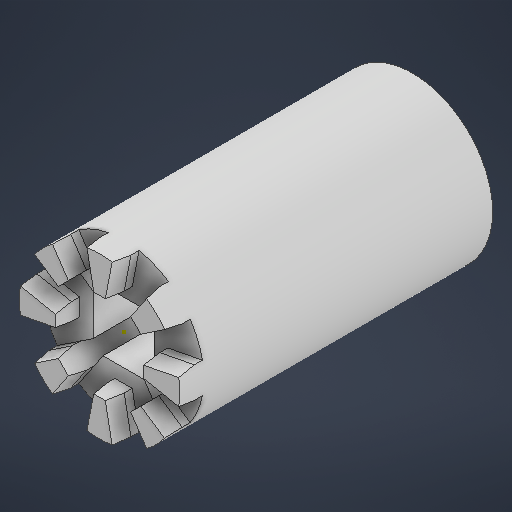
# Autodesk Inventor part: деталь вв
Saved by Autodesk Inventor 2025 (Build 290162000, 162)
## iProperties
Created: 2024-11-26
Part Number: деталь вв
Material: Типовые
Document SubType Name: Modeling
Designer: Phantom
Density: 1 g/cm^3
Appearance: По умолчанию
Author: Phantom
Autodesk Inventor part; units mm, degrees
ref_plane "YZ Plane" through (0, 0, 0) normal (1, 0, 0) x (0, 1, 0)
ref_plane "XZ Plane" through (0, 0, 0) normal (0, 1, 0) x (-1, 0, 0)
ref_plane "XY Plane" through (0, 0, 0) normal (0, 0, 1) x (1, 0, 0)
sketch "Эскиз1" plane through (0, 0, 0) normal (0, 0, 1) x (1, 0, 0)
  circle A0 centre (0, 0) radius 10
  line L0 (-3.8095, 3.8095) -> (3.8095, 3.8095)
  line L1 (3.8095, 3.8095) -> (3.8095, -3.8095)
  line L2 (3.8095, -3.8095) -> (-3.8095, -3.8095)
  line L3 (-3.8095, -3.8095) -> (-3.8095, 3.8095)
  line L4 (-3.8095, 3.8095) -> (3.8095, -3.8095) construction
  line L5 (3.8095, 3.8095) -> (-3.8095, -3.8095) construction
  dimension "d0" = 20
  constraints: 12 end point, 2 midpoint, 2 parallel, 1 centre point, 1 coincident, 1 horizontal, 1 perpendicular
  measures "d0" diameter of A0
extrude "Выдавливание1" add sketch "Эскиз1" along normal blind 36
sketch "Эскиз2" plane through (0, 0, 36) normal (0, 0, 1) x (1, 0, 0)
  line L0 (-3.8095, 3.8095) -> (3.8095, 3.8095) projected
  circle A0 centre (0, 0) radius 10 projected
  line L1 (9.8151, 1.914) -> (5.5, 1.0725)
  line L2 (5.5, -1.0775) -> (9.8135, -1.9225)
  line L3 (5.5, 0) -> (5.5, 1.0725)
  line L4 (5.5, 1.0725) -> (5.5, -1.0775)
  line L5 (5.587, 8.2937) -> (3.1307, 4.6475)
  line L6 (4.651, 3.1272) -> (8.2986, 5.5797)
  line L7 (3.8891, 3.8891) -> (3.1307, 4.6475)
  line L8 (3.1307, 4.6475) -> (4.651, 3.1272)
  line L9 (-1.914, 9.8151) -> (-1.0725, 5.5)
  line L10 (1.0775, 5.5) -> (1.9225, 9.8135)
  line L11 (0, 5.5) -> (-1.0725, 5.5)
  line L12 (-1.0725, 5.5) -> (1.0775, 5.5)
  line L13 (-8.2937, 5.587) -> (-4.6475, 3.1307)
  line L14 (-3.1272, 4.651) -> (-5.5797, 8.2986)
  line L15 (-3.8891, 3.8891) -> (-4.6475, 3.1307)
  line L16 (-4.6475, 3.1307) -> (-3.1272, 4.651)
  line L17 (-9.8151, -1.914) -> (-5.5, -1.0725)
  line L18 (-5.5, 1.0775) -> (-9.8135, 1.9225)
  line L19 (-5.5, 0) -> (-5.5, -1.0725)
  line L20 (-5.5, -1.0725) -> (-5.5, 1.0775)
  line L21 (-5.587, -8.2937) -> (-3.1307, -4.6475)
  line L22 (-4.651, -3.1272) -> (-8.2986, -5.5797)
  line L23 (-3.8891, -3.8891) -> (-3.1307, -4.6475)
  line L24 (-3.1307, -4.6475) -> (-4.651, -3.1272)
  line L25 (1.914, -9.8151) -> (1.0725, -5.5)
  line L26 (-1.0775, -5.5) -> (-1.9225, -9.8135)
  line L27 (0, -5.5) -> (1.0725, -5.5)
  line L28 (1.0725, -5.5) -> (-1.0775, -5.5)
  line L29 (8.2937, -5.587) -> (4.6475, -3.1307)
  line L30 (3.1272, -4.651) -> (5.5797, -8.2986)
  line L31 (3.8891, -3.8891) -> (4.6475, -3.1307)
  line L32 (4.6475, -3.1307) -> (3.1272, -4.651)
  dimension "d36" = 360
  constraints: 64 end point, 2 point on circle, 73 other
extrude "Выдавливание2" add sketch "Эскиз2" along normal blind 3 contours A0 L2 L4 L3 L1 | L6 L8 L7 L5 A0 | A0 L30 L32 L31 L29 | L10 L12 L11 L9 A0 | A0 L26 L28 L27 L25 | L14 L16 L15 L13 A0 | A0 L22 L24 L23 L21 | L18 L20 L19 L17 A0
chamfer "Фаска1" distance 2 angle 10 1 edges at (4.3588, 6.4706, 39) measured on face at (4.3588, 6.4706, 38.5)
chamfer "Фаска2" distance 2 angle 10 1 edges at (6.4748, 4.3535, 39) measured on face at (6.4748, 4.3535, 38.5)
chamfer "Фаска3" distance 2 angle 10 1 edges at (7.6576, 1.4932, 39) measured on face at (7.6576, 1.4932, 38.5)
chamfer "Фаска4" distance 2 angle 10 1 edges at (7.6567, -1.5, 39) measured on face at (7.6567, -1.5, 38.5)
chamfer "Фаска5" distance 2 angle 10 1 edges at (6.4706, -4.3588, 39) measured on face at (6.4706, -4.3588, 38.5)
chamfer "Фаска6" distance 2 angle 10 1 edges at (4.3535, -6.4748, 39) measured on face at (4.3535, -6.4748, 38.5)
chamfer "Фаска7" distance 2 angle 10 1 edges at (-1.5, -7.6567, 39) measured on face at (-1.5, -7.6567, 38.5)
chamfer "Фаска8" distance 2 angle 10 1 edges at (1.4932, -7.6576, 39) measured on face at (1.4932, -7.6576, 38.5)
chamfer "Фаска9" distance 2 angle 10 1 edges at (-6.4748, -4.3535, 39) measured on face at (-6.4748, -4.3535, 38.5)
chamfer "Фаска10" distance 2 angle 10 1 edges at (-4.3588, -6.4706, 39) measured on face at (-4.3588, -6.4706, 38.5)
chamfer "Фаска11" distance 2 angle 10 1 edges at (-7.6567, 1.5, 39) measured on face at (-7.6567, 1.5, 38.5)
chamfer "Фаска12" distance 2 angle 10 1 edges at (-7.6576, -1.4932, 39) measured on face at (-7.6576, -1.4932, 38.5)
chamfer "Фаска13" distance 2 angle 10 1 edges at (-4.3535, 6.4748, 39) measured on face at (-4.3535, 6.4748, 38.5)
chamfer "Фаска14" distance 2 angle 10 1 edges at (-6.4706, 4.3588, 39) measured on face at (-6.4706, 4.3588, 38.5)
chamfer "Фаска15" distance 2 angle 10 1 edges at (1.5, 7.6567, 39) measured on face at (1.5, 7.6567, 38.5)
chamfer "Фаска16" distance 2 angle 10 1 edges at (-1.4932, 7.6576, 39) measured on face at (-1.4932, 7.6576, 38.5)
sketch "Эскиз3" plane through (0, 0, 36) normal (0, 0, 1) x (1, 0, 0)
  point P0 (0, 0)
sketch "Эскиз4" plane through (0, 0, 39) normal (0, 0, 1) x (1, 0, 0)
  line L0 (-3.8095, 3.8095) -> (3.8095, 3.8095) projected
  line L1 (3.8095, 3.8095) -> (4.5166, 4.5166)
  line L2 (5.587, 8.2937) -> (3.1307, 4.6475) projected
  line L3 (4.651, 3.1272) -> (8.2986, 5.5797) projected
  line L4 (4.5166, 4.5166) -> (3.6359, 5.3974)
  line L5 (3.1307, 4.6475) -> (5.587, 8.2937) projected
  line L6 (4.5166, 4.5166) -> (5.4015, 3.6318)
  line L7 (5.4015, 3.6318) -> (3.3919, 2.2806)
  line L8 (3.6359, 5.3974) -> (2.2483, 3.3376)
  line L9 (2.2483, 3.3376) -> (3.3919, 2.2806)
  line L10 (-3.8095, 3.8095) -> (-4.5166, 4.5166)
  line L11 (-4.5166, 4.5166) -> (-5.3974, 3.6359)
  line L12 (-4.5166, 4.5166) -> (-3.6318, 5.4015)
  line L13 (-3.6318, 5.4015) -> (-2.2806, 3.3919)
  line L14 (-5.3974, 3.6359) -> (-3.3376, 2.2483)
  line L15 (-3.3376, 2.2483) -> (-2.2806, 3.3919)
  line L16 (-3.8095, -3.8095) -> (-4.5166, -4.5166)
  line L17 (-4.5166, -4.5166) -> (-3.6359, -5.3974)
  line L18 (-4.5166, -4.5166) -> (-5.4015, -3.6318)
  line L19 (-5.4015, -3.6318) -> (-3.3919, -2.2806)
  line L20 (-3.6359, -5.3974) -> (-2.2483, -3.3376)
  line L21 (-2.2483, -3.3376) -> (-3.3919, -2.2806)
  line L22 (3.8095, -3.8095) -> (4.5166, -4.5166)
  line L23 (4.5166, -4.5166) -> (5.3974, -3.6359)
  line L24 (4.5166, -4.5166) -> (3.6318, -5.4015)
  line L25 (3.6318, -5.4015) -> (2.2806, -3.3919)
  line L26 (5.3974, -3.6359) -> (3.3376, -2.2483)
  line L27 (3.3376, -2.2483) -> (2.2806, -3.3919)
  point P0 (0, 0)
  dimension "d86" = 1
  dimension "d89" = 360
  constraints: 48 end point, 7 point on line, 49 other
  measures "d86" distance of L0.end L1.end
extrude "Выдавливание3" cut sketch "Эскиз4" against normal through all
